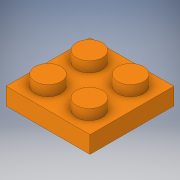
# Autodesk Inventor part: 2x2 short orange pegged
Saved by Autodesk Inventor 2017 (Build 210142000, 142)
## iProperties
Created: 2018-05-10
Part Number: 2x2 short orange pegged
Material: ABS Plastic
Document SubType Name: Modeling
Designer: 20000650
Density: 1.06 g/cm^3
Appearance: Orange
Author: 20000650
Autodesk Inventor part; units mm, degrees
ref_plane "YZ Plane" through (0, 0, 0) normal (1, 0, 0) x (0, 1, 0)
ref_plane "XZ Plane" through (0, 0, 0) normal (0, 1, 0) x (-1, 0, 0)
ref_plane "XY Plane" through (0, 0, 0) normal (0, 0, 1) x (1, 0, 0)
sketch "Sketch1" plane through (0, 0, 0) normal (0, 1, 0) x (-1, 0, 0)
  line L0 (0, 0) -> (0, -15.8369)
  line L1 (0, -15.8369) -> (15.8369, -15.8369)
  line L2 (15.8369, -15.8369) -> (15.8369, 0)
  line L3 (15.8369, 0) -> (0, 0)
  dimension "d0" = 15.8369
  dimension "d1" = 15.8369
  dimension "d2" = 15.8369
  constraints: 8 end point, 2 perpendicular, 1 vertical
  measures "d0" distance of L0.start L0.end
  measures "d1" distance of L0.end L1.end
  measures "d2" distance of L1.end L2.end
extrude "Extrusion1" add sketch "Sketch1" along normal blind 3.236
sketch "Sketch2" plane through (0, 3.236, 0) normal (0, 1, 0) x (1, 0, 0)
  line L0 (-15.8369, 15.8369) -> (-15.8369, 0) projected
  line L1 (-15.8369, 0) -> (0, 15.8369)
  line L2 (0, 15.8369) -> (-15.8369, 15.8369)
  line L3 (-15.8369, 15.8369) -> (0, 0)
  line L4 (-7.9185, 7.9185) -> (0, 7.9185)
  line L5 (0, 7.9185) -> (-15.8369, 7.9185)
  line L6 (-7.9185, 7.9185) -> (-7.9185, 15.8369)
  line L7 (0, 15.8369) -> (-15.8369, 15.8369) projected
  line L8 (-7.9185, 0) -> (-7.9185, 7.9185)
  line L9 (-7.9185, 0) -> (-15.8369, 7.9185)
  line L10 (-15.8369, 7.9185) -> (-7.9185, 15.8369)
  line L11 (0, 7.9185) -> (-7.9185, 15.8369)
  line L12 (-7.9185, 0) -> (0, 7.9185)
  circle A0 centre (-11.8777, 3.9592) radius 2.4498
  dimension "d5" = 4.8997
  constraints: 22 end point, 5 perpendicular, 4 midpoint, 1 centre point, 1 horizontal, 1 point on line
  measures "d5" diameter of A0
extrude "Extrusion2" add sketch "Sketch2" along normal blind 1.9837 contours A0 L1 L9 | L9 L1 A0 | L1 L9 A0 | A0 L9 L1
pattern_linear "Rectangular Pattern1" count 2 spacing 7.7978 along (1, 0, 0) count 2 spacing 7.7978 along (0, 0, -1) of "Extrusion2"
shell "Shell1" thickness 1.4732 removed faces 1 at (-5.279, 0, -10.5579)
sketch "Sketch3" plane through (0, 0, 0) normal (0, 1, 0) x (-1, 0, 0)
  circle A0 centre (4.0799, -3.9592) radius 2.4498 construction
  circle A1 centre (11.8777, -11.757) radius 2.4498 construction
  line L0 (4.0799, -3.9592) -> (11.8777, -11.757) construction
  circle A2 centre (7.9788, -7.8581) radius 3.064
  circle A3 centre (7.9788, -7.8581) radius 2.4498
  point P0 (0, 0)
  dimension "d15" = 4.8997
  constraints: 2 centre point, 2 end point, 1 coincident, 1 midpoint
  measures "d15" diameter of A3
extrude "Extrusion3" add sketch "Sketch3" along normal up to surface (1.7628 mm away)
body "Solid1"
